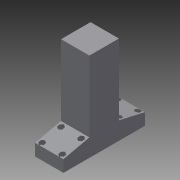
# Autodesk Inventor part: Rotational Arm
Saved by Autodesk Inventor 2015 SP1 (Build 190203100, 203)
## iProperties
Created: 2015-02-24
Part Number: Rotational Arm
Material: Generic
Document SubType Name: Modeling
Designer: Andrew
Density: 1 g/cm^3
Appearance: Default
Author: Andrew
Autodesk Inventor part; units mm, degrees
ref_plane "YZ Plane" through (0, 0, 0) normal (1, 0, 0) x (0, 1, 0)
ref_plane "XZ Plane" through (0, 0, 0) normal (0, 1, 0) x (-1, 0, 0)
sketch "Sketch1" plane through (0, 0, 0) normal (1, 0, 0) x (0, 1, 0)
  line L0 (0, 69) -> (0, -69)
  line L1 (0, -69) -> (20, -69)
  line L2 (20, -69) -> (30, -25)
  line L3 (30, -25) -> (150, -25)
  line L4 (150, -25) -> (150, 25)
  line L5 (150, 25) -> (30, 25)
  line L6 (30, 25) -> (20, 69)
  line L7 (20, 69) -> (0, 69)
  line L8 (-30, 0) -> (180, 0) projected
  line L9 (0, 96.6) -> (0, -96.6) projected
  point P0 (0, 0)
  dimension "d0" = 138
  dimension "d1" = 150
  dimension "d2" = 50
  dimension "d3" = 120
  dimension "d4" = 20
  constraints: 16 end point, 3 perpendicular, 2 parallel, 1 collinear, 1 vertical, 3 other
  measures "d0" distance between parallel lines of L1 L7
  measures "d1" distance between parallel lines of L0 L4
  measures "d2" distance between parallel lines of L5 L3
  measures "d3" distance of L2.end L3.end
  measures "d4" distance of L0.end L1.end
extrude "Extrusion1" add sketch "Sketch1" along normal mid plane 48
sketch "Sketch2" plane through (-24, 0, -69) normal (0, -1, 0) x (1, 0, 0)
  circle A0 centre (7, 5) radius 2.75
  circle A1 centre (7, 37) radius 2.75
  circle A2 centre (41, 5) radius 2.75
  circle A3 centre (41, 37) radius 2.75
  circle A4 centre (7, 101) radius 2.75
  circle A5 centre (7, 133) radius 2.75
  circle A6 centre (41, 101) radius 2.75
  circle A7 centre (41, 133) radius 2.75
  line L0 (-9.6, 69) -> (57.6, 69) projected
  line L1 (24, 165.6) -> (24, -27.6) projected
  line L2 (7, 5) -> (7, 37) construction
  line L3 (0, 0) -> (48, 0) projected
  point P0 (24, 69)
  dimension "d7" = 32
  dimension "d8" = 5.5
  dimension "d9" = 5
  dimension "d10" = 34
  constraints: 8 centre point, 2 end point, 1 equal radius, 1 vertical, 6 other
  measures "d7" distance of L2.end L2.start
  measures "d8" diameter of A0
  measures "d9" distance from line of L3 L2.start
  measures "d10" distance of A2.centre L2.start
extrude "Extrusion2" cut sketch "Sketch2" against normal up to next
ref_plane "Work Plane1" through (-24, 15, -69) normal (0, -1, 0) x (1, 0, 0)
sketch "Sketch3" plane through (-24, 15, -69) normal (0, -1, 0) x (1, 0, 0)
  circle A0 centre (41, 5) radius 2.75 projected
  circle A1 centre (7, 5) radius 2.75 projected
  circle A2 centre (7, 37) radius 2.75 projected
  circle A3 centre (41, 37) radius 2.75 projected
  line L0 (0, 44) -> (48, 44) projected
  line L1 (48, 0) -> (48, 44) projected
  line L2 (0, 0) -> (48, 0) projected
  line L3 (0, 44) -> (0, 0) projected
  circle A4 centre (41, 101) radius 2.75 projected
  circle A5 centre (7, 101) radius 2.75 projected
  circle A6 centre (7, 133) radius 2.75 projected
  circle A7 centre (41, 133) radius 2.75 projected
  line L4 (0, 138) -> (48, 138) projected
  line L5 (48, 94) -> (48, 138) projected
  line L6 (0, 94) -> (48, 94) projected
  line L7 (0, 138) -> (0, 94) projected
  circle A8 centre (7, 133) radius 2.75 construction
  line L8 (7, 133) -> (41, 101) construction
  circle A9 centre (41, 133) radius 2.75 construction
  line L9 (7, 101) -> (41, 133) construction
  circle A10 centre (41, 5) radius 2.75 construction
  line L10 (7, 37) -> (41, 5) construction
  line L11 (7, 5) -> (41, 37) construction
  line L12 (7, 128) -> (2.6699, 130.5)
  line L13 (2.6699, 130.5) -> (2.6699, 135.5)
  line L14 (2.6699, 135.5) -> (7, 138)
  line L15 (7, 138) -> (11.3301, 135.5)
  line L16 (11.3301, 135.5) -> (11.3301, 130.5)
  line L17 (11.3301, 130.5) -> (7, 128)
  line L18 (41, 128) -> (36.6699, 130.5)
  line L19 (36.6699, 130.5) -> (36.6699, 135.5)
  line L20 (36.6699, 135.5) -> (41, 138)
  line L21 (41, 138) -> (45.3301, 135.5)
  line L22 (45.3301, 135.5) -> (45.3301, 130.5)
  line L23 (45.3301, 130.5) -> (41, 128)
  circle A11 centre (41, 101) radius 2.75 projected
  line L24 (41, 96) -> (36.6699, 98.5)
  line L25 (36.6699, 98.5) -> (36.6699, 103.5)
  line L26 (36.6699, 103.5) -> (41, 106)
  line L27 (41, 106) -> (45.3301, 103.5)
  line L28 (45.3301, 103.5) -> (45.3301, 98.5)
  line L29 (45.3301, 98.5) -> (41, 96)
  line L30 (7, 96) -> (2.6699, 98.5)
  line L31 (2.6699, 98.5) -> (2.6699, 103.5)
  line L32 (2.6699, 103.5) -> (7, 106)
  line L33 (7, 106) -> (11.3301, 103.5)
  line L34 (11.3301, 103.5) -> (11.3301, 98.5)
  line L35 (11.3301, 98.5) -> (7, 96)
  line L36 (-9.6, 69) -> (57.6, 69) projected
  line L37 (7, 32) -> (2.6699, 34.5)
  line L38 (2.6699, 34.5) -> (2.6699, 39.5)
  line L39 (2.6699, 39.5) -> (7, 42)
  line L40 (7, 42) -> (11.3301, 39.5)
  line L41 (11.3301, 39.5) -> (11.3301, 34.5)
  line L42 (11.3301, 34.5) -> (7, 32)
  line L43 (7, 0) -> (2.6699, 2.5)
  line L44 (2.6699, 2.5) -> (2.6699, 7.5)
  line L45 (2.6699, 7.5) -> (7, 10)
  line L46 (7, 10) -> (11.3301, 7.5)
  line L47 (11.3301, 7.5) -> (11.3301, 2.5)
  line L48 (11.3301, 2.5) -> (7, 0)
  line L49 (41, 0) -> (36.6699, 2.5)
  line L50 (36.6699, 2.5) -> (36.6699, 7.5)
  line L51 (36.6699, 7.5) -> (41, 10)
  line L52 (41, 10) -> (45.3301, 7.5)
  line L53 (45.3301, 7.5) -> (45.3301, 2.5)
  line L54 (45.3301, 2.5) -> (41, 0)
  line L55 (41, 32) -> (36.6699, 34.5)
  line L56 (36.6699, 34.5) -> (36.6699, 39.5)
  line L57 (36.6699, 39.5) -> (41, 42)
  line L58 (41, 42) -> (45.3301, 39.5)
  line L59 (45.3301, 39.5) -> (45.3301, 34.5)
  line L60 (45.3301, 34.5) -> (41, 32)
  point P0 (24, 69)
  dimension "d14" = 5
  constraints: 104 end point, 8 coincident, 5 parallel, 2 collinear, 108 other
  measures "d14" distance of L32.end L33.end
extrude "Extrusion3" cut sketch "Sketch3" against normal up to next contours L43 L44 L45 L46 L47 L48 | L49 L50 L51 L52 L53 L54 | L21 L22 L23 L18 L19 L20 | L15 L16 L17 L12 L13 L14 | L24 L25 L26 L27 L28 L29 | L30 L31 L32 L33 L34 L35 | L37 L38 L39 L40 L41 L42 | L55 L56 L57 L58 L59 L60
body "Solid1"
